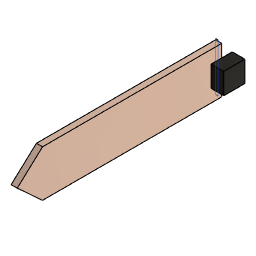
_ capacitive soil humidity sensor v5 (Autodesk Fusion 360 design; units mm, degrees)
Autodesk Fusion 360 part; units mm, degrees
sketch "Sketch1" plane through (0, 0, 0) normal (1, 0, 0) x (0, 0, -1)
  line L0 (0, 0) -> (22, 0)
  line L1 (22, 0) -> (22, -97)
  line L2 (22, -97) -> (0, -97)
  line L3 (0, -97) -> (0, 0)
  line L4 (14, -97) -> (8, -97)
  line L5 (11, 0) -> (11, -97) construction
  line L6 (11, -97) -> (0, -85)
  line L7 (11, -97) -> (22, -85)
  point P0 (11, -97)
  dimension "d46" = 97
  dimension "d47" = 22
  dimension "d2" = 12
  constraint horizontal L0
  constraint vertical L1
  constraint horizontal L2
  constraint vertical L3
  constraint coincident L0.start L3.end
  constraint horizontal L4
  constraint collinear L2 L4
  constraint midpoint L4 P0
  constraint midpoint L2 P0
  constraint midpoint L0 L5.start
  constraint coincident P0 L5.end
  constraint coincident L3 L6.end
  constraint symmetric L5 P0 L6.start
  constraint symmetric L5 L6.end L7.end
  measures "d46" distance of L0.start L2.end
  measures "d47" distance of L0.start L0.end
  measures "d2" distance of L2.end L6.end
extrude "Extrude1" add sketch "Sketch1" along normal blind 2.9 contours L0 L1 L3 L6 L7 makes body 1
ref_plane "WorkPlane1" through (2.9, -48.5, -11) normal (1, 0, 0) x (0, 0, -1)
sketch "Sketch2" plane through (2.9, -30, -10) normal (1, 0, 0) x (0, 0, -1)
  line L0 (12, 30) -> (-10, 30)
  line L1 (1, -67) -> (1, 30) construction
  line L2 (6, 35) -> (-4, 35)
  line L3 (-4, 35) -> (-4, 25)
  line L4 (-4, 25) -> (6, 25)
  line L5 (6, 25) -> (6, 35)
  line L6 (6, 35) -> (-4, 25) construction
  line L7 (-4, 35) -> (6, 25) construction
  point P0 (1, -67)
  point P1 (1, 30)
  dimension "d4" = 10
  dimension "d5" = 10
  constraint coincident P0 L1.start
  constraint midpoint L0 P1
  constraint perpendicular L2 L3
  constraint parallel L2 L4
  constraint parallel L3 L5
  constraint horizontal L2
  constraint coincident L6 P1
  constraint coincident L7 P1
  constraint coincident P1 L1.end
  measures "d4" distance of L2.end L3.end
  measures "d5" distance of L3.end L4.end
extrude "Extrude2" add sketch "Sketch2" along normal blind 6 separate body makes body 2
sketch "Sketch6" plane through (0, 0, 0) normal (0, 1, 0) x (-1, 0, 0)
  line L0 (0, -22) -> (0, 0)
  line L1 (0, 0) -> (-2.9, 0)
  line L2 (-2.9, 0) -> (-2.9, -22)
  line L3 (-2.9, -22) -> (0, -22)
  line L4 (-1.2, 0.5) -> (0, 0.5)
  line L5 (0, 0.5) -> (0, -22.5)
  line L6 (0, -22.5) -> (-1.2, -22.5)
  line L7 (-1.2, -22.5) -> (-1.2, 0.5)
  dimension "d6" = 0.5
  dimension "d7" = 0.5
  constraint horizontal L4
  constraint vertical L5
  constraint horizontal L6
  constraint vertical L7
  measures "d6" distance of L1 L4
  measures "d7" distance of L3 L6
